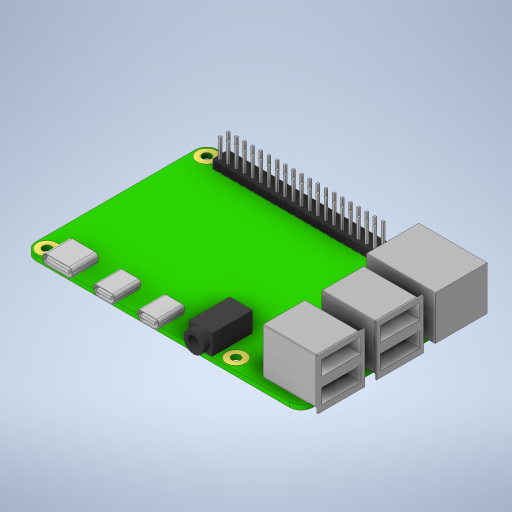
# Autodesk Inventor part: raspberry
Saved by Autodesk Inventor 2023.1 (Build 271208000, 208)
## iProperties
Created: 2022-05-23
Part Number: raspberry
Material: 일반
Document SubType Name: Modeling
Designer: fly01
Density: 1 g/cm^3
Appearance: 기본값
Author: fly01
Autodesk Inventor part; units mm, degrees
ref_plane "YZ Plane" through (0, 0, 0) normal (1, 0, 0) x (0, 1, 0)
ref_plane "XZ Plane" through (0, 0, 0) normal (0, 1, 0) x (-1, 0, 0)
ref_plane "XY Plane" through (0, 0, 0) normal (0, 0, 1) x (1, 0, 0)
sketch "스케치1" plane through (0, 0, 0) normal (0, 0, 1) x (1, 0, 0)
  line L0 (-39, 28) -> (39, 28)
  line L1 (42.5, 24.5) -> (42.5, -24.5)
  line L2 (39, -28) -> (-39, -28)
  line L3 (-42.5, -24.5) -> (-42.5, 24.5)
  line L4 (-42.5, 28) -> (42.5, -28) construction
  line L5 (42.5, 28) -> (-42.5, -28) construction
  circle A0 centre (-39, 24.5) radius 1.35
  circle A1 centre (-39, 24.5) radius 3
  line L6 (0, 0) -> (24.8557, 0)
  arc A2 (-39, 28) -> (-42.5, 24.5) centre (-39, 24.5) ccw
  circle A3 centre (19, 24.5) radius 3
  circle A4 centre (19, 24.5) radius 1.35
  circle A5 centre (-39, -24.5) radius 1.35
  circle A6 centre (-39, -24.5) radius 3
  circle A7 centre (19, -24.5) radius 3
  circle A8 centre (19, -24.5) radius 1.35
  arc A9 (-42.5, -24.5) -> (-39, -28) centre (-39, -24.5) ccw
  arc A10 (39, -28) -> (42.5, -24.5) centre (39, -24.5) ccw
  arc A11 (42.5, 24.5) -> (39, 28) centre (39, 24.5) ccw
  dimension "d0" = 85
  dimension "d1" = 56
  dimension "d2" = 2.7
  dimension "d3" = 6
  dimension "d5" = 3.5
  dimension "d6" = 3.5
  dimension "d7" = 3.5
  dimension "d10" = 58
  dimension "d15" = 3.5
  constraints: 14 end point, 12 centre point, 8 point on circle, 8 point on line, 8 tangent, 4 coincident, 4 symmetric about line, 3 horizontal, 2 equal radius, 2 midpoint, 2 parallel, 1 perpendicular, 8 other
  measures "d0" distance of L4.start L5.start
  measures "d1" distance of L5.start L4.end
  measures "d2" diameter of A0
  measures "d3" diameter of A1
  measures "d5" distance from line of L0 A0.centre
  measures "d6" distance from line of L3 A0.centre
  measures "d7" radius of A2
  measures "d10" distance of A1.centre A3.centre
  measures "d15" radius of A9
extrude "돌출1" add sketch "스케치1" against normal blind 1.5 contours L0 A11 L1 A10 L2 A9 L3 A2
extrude "돌출2" add sketch "스케치1" against normal blind 1.51 contours A1 | A3 | A6 | A7
sketch "스케치2" plane through (0, 0, -1.5) normal (0, 0, -1) x (-1, 0, 0)
  line L0 (-24.8, -25.75) -> (-45.8, -25.75)
  line L1 (-45.8, -25.75) -> (-45.8, -9.75)
  line L2 (-45.8, -9.75) -> (-24.8, -9.75)
  line L3 (-24.8, -9.75) -> (-24.8, -25.75)
  line L4 (-24.8, -25.75) -> (-45.8, -9.75) construction
  line L5 (-45.8, -25.75) -> (-24.8, -9.75) construction
  line L6 (-28.3, -5.5) -> (-45.8, -5.5)
  line L7 (-45.8, -5.5) -> (-45.8, 7.5)
  line L8 (-45.8, 7.5) -> (-28.3, 7.5)
  line L9 (-28.3, 7.5) -> (-28.3, -5.5)
  line L10 (-28.3, -5.5) -> (-45.8, 7.5) construction
  line L11 (-45.8, -5.5) -> (-28.3, 7.5) construction
  line L12 (-28.3, 12.5) -> (-45.8, 12.5)
  line L13 (-45.8, 12.5) -> (-45.8, 25.5)
  line L14 (-45.8, 25.5) -> (-28.3, 25.5)
  line L15 (-28.3, 25.5) -> (-28.3, 12.5)
  line L16 (-28.3, 12.5) -> (-45.8, 25.5) construction
  line L17 (-45.8, 12.5) -> (-28.3, 25.5) construction
  line L18 (39, 28) -> (-39, 28) projected
  line L19 (-42.5, 24.5) -> (-42.5, -24.5) projected
  point P0 (0, 0)
  point P1 (-35.3, -17.75)
  point P2 (-37.05, 1)
  point P3 (-37.05, 19)
  dimension "d20" = 45.75
  dimension "d21" = 27
  dimension "d22" = 9
  dimension "d23" = 16
  dimension "d24" = 21
  dimension "d25" = 13
  dimension "d26" = 17.5
  dimension "d27" = 13
  dimension "d28" = 17.5
  dimension "d29" = 3.3
  constraints: 36 end point, 6 midpoint, 6 parallel, 3 horizontal, 3 perpendicular, 2 point on line
  measures "d20" distance from line of L18 point (-35.3, -17.75)
  measures "d21" distance from line of L18 point (-37.05, 1)
  measures "d22" distance from line of L18 point (-37.05, 19)
  measures "d23" distance between parallel lines of L2 L0
  measures "d24" distance of L0.start L0.end
  measures "d25" distance of L6.end L7.end
  measures "d26" distance of L6.start L6.end
  measures "d27" distance of L12.end L13.end
  measures "d28" distance of L12.start L12.end
  measures "d29" distance between parallel lines of L19 L13
extrude "돌출3" add sketch "스케치2" along normal blind 13.5 contours L0 L1 L2 L3
extrude "돌출4" add sketch "스케치2" along normal blind 14 contours L6 L19 L8 L9 | L6 L7 L8 L19 | L12 L13 L14 L15
sketch "스케치3" plane through (45.8, 12.5, -1.5) normal (1, 0, 0) x (0, 0, -1)
  line L0 (0, 13) -> (0, 0) projected
  line L1 (0, 0) -> (14, 0) projected
  line L2 (14, 13) -> (14, 0) projected
  line L3 (0, 13) -> (14, 13) projected
  line L4 (0, -5) -> (0, -18) projected
  line L5 (0, -18) -> (14, -18) projected
  line L6 (14, -5) -> (14, -18) projected
  line L7 (0, -5) -> (14, -5) projected
  line L8 (14.7, -0.7) -> (-0.7, -0.7)
  line L9 (-0.7, -0.7) -> (-0.7, 13.7)
  line L10 (-0.7, 13.7) -> (14.7, 13.7)
  line L11 (14.7, 13.7) -> (14.7, -0.7)
  line L12 (14.7, -18.7) -> (-0.7, -18.7)
  line L13 (-0.7, -18.7) -> (-0.7, -4.3)
  line L14 (-0.7, -4.3) -> (14.7, -4.3)
  line L15 (14.7, -4.3) -> (14.7, -18.7)
  point P0 (-1.5, -12.5)
  dimension "d34" = 0.7
  dimension "d35" = 0.7
  constraints: 16 end point, 6 other
  measures "d34" distance between parallel lines of L2 L11
  measures "d35" distance between parallel lines of L6 L15
extrude "돌출5" add sketch "스케치3" against normal blind 0.3 contours L3 L2 L1 L0 | L7 L6 L5 L4 | L8 L9 L10 L11 | L12 L13 L14 L15
fillet "모깎기1" radius 0.2 8 edges at (36.9, 25.5, -15.5) (36.9, 12.5, -15.5) (36.9, 7.5, -15.5) (36.9, -5.5, -15.5) (44, -5.5, -1.5) (44, 7.5, -1.5) (44, 12.5, -1.5) (43.9271, 25.5, -1.5)
fillet "모깎기2" radius 1 16 edges at (45.5, -5.4414, -15.4414) (45.5, -5.5, -8.5) (45.5, -5.4414, -1.5586) (45.5, 1, -1.5) (45.5, 7.4414, -1.5586) (45.5, 7.5, -8.5) (45.5, 7.4414, -15.4414) (45.5, 1, -15.5) (45.5, 12.5586, -15.4414) (45.5, 12.5, -8.5) (45.5, 12.5586, -1.5586) (45.5, 19, -1.5) (45.5, 25.4414, -1.5586) (45.5, 25.5, -8.5) (45.5, 25.4414, -15.4414) (45.5, 19, -15.5)
sketch "스케치4" plane through (0, 0, -1.5) normal (0, 0, -1) x (-1, 0, 0)
  line L0 (35.8, 21) -> (26.8, 21)
  line L1 (26.8, 21) -> (26.8, 29)
  line L2 (26.8, 29) -> (35.8, 29)
  line L3 (35.8, 29) -> (35.8, 21)
  line L4 (35.8, 21) -> (26.8, 29) construction
  line L5 (26.8, 21) -> (35.8, 29) construction
  circle A0 centre (39, 24.5) radius 1.35 projected
  line L6 (39, 28) -> (-39, 28) projected
  point P0 (0, 0)
  point P1 (31.3, 25)
  dimension "d40" = 9
  dimension "d41" = 8
  dimension "d42" = 7.7
  dimension "d43" = 1
  constraints: 12 end point, 2 midpoint, 2 parallel, 1 horizontal, 1 perpendicular
  measures "d40" distance of L1.end L2.end
  measures "d41" distance of L0.end L1.end
  measures "d42" horizontal distance of point (31.3, 25) A0.centre
  measures "d43" distance between parallel lines of L6 L2
extrude "돌출6" add sketch "스케치4" along normal blind 3 contours L0 L1 L6 L3 | L6 L1 L2 L3
sketch "스케치5" plane through (-35.8, 29, -1.5) normal (0, 1, 0) x (1, 0, 0)
  line L0 (0, 0) -> (0, 3) projected
  line L1 (1, 3) -> (8, 3)
  line L2 (9, 2) -> (9, 1)
  line L3 (8, 0) -> (1, 0)
  line L4 (0, 1) -> (0, 2)
  arc A0 (1, 3) -> (0, 2) centre (1, 2) ccw
  arc A1 (0, 1) -> (1, 0) centre (1, 1) ccw
  arc A2 (8, 0) -> (9, 1) centre (8, 1) ccw
  arc A3 (9, 2) -> (8, 3) centre (8, 2) ccw
  line L5 (0, 3) -> (9, 3)
  line L6 (9, 3) -> (9, 0)
  line L7 (9, 0) -> (0, 0)
  line L8 (0, 0) -> (0, 3)
  line L9 (1, 2) -> (8, 2)
  line L10 (8, 2) -> (8, 1)
  line L11 (8, 1) -> (1, 1)
  line L12 (1, 1) -> (1, 2)
  line L13 (8, 2.8) -> (1, 2.8)
  arc A4 (1, 2.8) -> (0.2, 2) centre (1, 2) ccw
  line L14 (0.2, 2) -> (0.2, 1)
  arc A5 (0.2, 1) -> (1, 0.2) centre (1, 1) ccw
  line L15 (1, 0.2) -> (8, 0.2)
  arc A6 (8, 0.2) -> (8.8, 1) centre (8, 1) ccw
  line L16 (8.8, 1) -> (8.8, 2)
  arc A7 (8.8, 2) -> (8, 2.8) centre (8, 2) ccw
  point P0 (35.8, -1.5)
  point P1 (8, 0)
  point P2 (9, 1)
  point P3 (9, 2)
  point P4 (8, 3)
  point P5 (1, 3)
  point P6 (0, 2)
  point P7 (1, 0)
  point P8 (0, 1)
  dimension "d46" = 1
  dimension "d49" = 0.2
  constraints: 32 end point, 16 point on circle, 8 centre point, 8 parallel, 8 tangent, 4 perpendicular, 4 point on line, 3 equal radius, 3 horizontal, 7 other
  measures "d46" radius of A0
  measures "d49" distance between parallel lines of L1 L13
extrude "돌출7" cut sketch "스케치5" against normal blind 8 contours L0 A1 L7 | L0 L5 A0 | A2 L6 L7 | L5 L6 A3
extrude "돌출8" cut sketch "스케치5" against normal blind 7 contours A7 L16 A6 L15 A5 L14 A4 L13
sketch "스케치6" plane through (0, 0, -1.5) normal (0, 0, -1) x (-1, 0, 0)
  line L0 (19.75, 21.5) -> (13.25, 21.5)
  line L1 (13.25, 21.5) -> (13.25, 29.5)
  line L2 (13.25, 29.5) -> (19.75, 29.5)
  line L3 (19.75, 29.5) -> (19.75, 21.5)
  line L4 (19.75, 21.5) -> (13.25, 29.5) construction
  line L5 (13.25, 21.5) -> (19.75, 29.5) construction
  line L6 (34.8, 21) -> (27.8, 21) projected
  line L7 (31.3, 21) -> (31.3, 13.0642)
  line L8 (27.8, 28) -> (-39, 28) projected
  point P0 (0, 0)
  point P1 (16.5, 25.5)
  dimension "d52" = 14.8
  dimension "d53" = 1.5
  dimension "d54" = 8
  dimension "d55" = 6.5
  constraints: 14 end point, 3 midpoint, 2 parallel, 1 horizontal, 1 perpendicular, 1 vertical
  measures "d52" distance from line of L7 point (16.5, 25.5)
  measures "d53" distance between parallel lines of L8 L2
  measures "d54" distance of L0.end L1.end
  measures "d55" distance of L0.start L0.end
extrude "돌출9" add sketch "스케치6" along normal blind 3
sketch "스케치7" plane through (-19.75, 29.5, -1.5) normal (0, 1, 0) x (1, 0, 0)
  line L0 (0, 0) -> (6.5, 0) projected
  line L1 (6.5, 0) -> (6.5, 3) projected
  line L2 (0, 3) -> (6.5, 3) projected
  line L3 (0, 0) -> (0, 3) projected
  line L4 (0, 0) -> (0, 3) projected
  line L5 (0.7, 3) -> (5.8, 3)
  line L6 (6.5, 2.3) -> (6.5, 1.6348)
  line L7 (5.4261, 0) -> (1.0739, 0)
  line L8 (0, 1.6348) -> (0, 2.3)
  line L9 (0.0501, 1.3748) -> (0.424, 0.44)
  line L10 (6.4499, 1.3748) -> (6.076, 0.44)
  arc A0 (0.424, 0.44) -> (1.0739, 0) centre (1.0739, 0.7) ccw
  arc A1 (0, 1.6348) -> (0.0501, 1.3748) centre (0.7, 1.6348) ccw
  arc A2 (5.4261, 0) -> (6.076, 0.44) centre (5.4261, 0.7) ccw
  arc A3 (6.4499, 1.3748) -> (6.5, 1.6348) centre (5.8, 1.6348) ccw
  arc A4 (6.5, 2.3) -> (5.8, 3) centre (5.8, 2.3) ccw
  arc A5 (0.7, 3) -> (0, 2.3) centre (0.7, 2.3) ccw
  line L11 (0.2, 2.3) -> (0.2, 1.6348)
  arc A6 (0.2, 1.6348) -> (0.2358, 1.4491) centre (0.7, 1.6348) ccw
  line L12 (0.2358, 1.4491) -> (0.6097, 0.5143)
  arc A7 (0.6097, 0.5143) -> (1.0739, 0.2) centre (1.0739, 0.7) ccw
  line L13 (1.0739, 0.2) -> (5.4261, 0.2)
  arc A8 (5.4261, 0.2) -> (5.8903, 0.5143) centre (5.4261, 0.7) ccw
  line L14 (5.8903, 0.5143) -> (6.2642, 1.4491)
  arc A9 (6.2642, 1.4491) -> (6.3, 1.6348) centre (5.8, 1.6348) ccw
  line L15 (6.3, 1.6348) -> (6.3, 2.3)
  arc A10 (6.3, 2.3) -> (5.8, 2.8) centre (5.8, 2.3) ccw
  line L16 (5.8, 2.8) -> (0.7, 2.8)
  arc A11 (0.7, 2.8) -> (0.2, 2.3) centre (0.7, 2.3) ccw
  line L17 (1.0733, 1.9674) -> (5.3358, 1.9674)
  line L18 (5.3358, 1.9674) -> (5.3358, 1.2025)
  line L19 (5.3358, 1.2025) -> (1.0733, 1.2025)
  line L20 (1.0733, 1.2025) -> (1.0733, 1.9674)
  point P0 (19.75, -1.5)
  point P1 (0, 1.5)
  point P2 (0.6, 0)
  point P3 (6.5, 1.5)
  point P4 (5.9, 0)
  point P5 (0, 2.3)
  point P6 (0.7, 3)
  point P7 (0, 1.6348)
  point P8 (6.5, 1.6348)
  point P9 (5.8, 3)
  dimension "d58" = 1.5
  dimension "d59" = 0.6
  dimension "d60" = 1.5
  dimension "d61" = 0.6
  dimension "d62" = 0.7
  dimension "d63" = 0.2
  constraints: 32 end point, 24 point on circle, 14 point on line, 12 centre point, 12 tangent, 6 parallel, 5 equal radius, 3 perpendicular, 2 horizontal, 11 other
  measures "d58" distance of point (0, 1.5) point (0, 0)
  measures "d59" distance of point (0.6, 0) point (0, 0)
  measures "d60" distance of point (6.5, 1.5) L0.end
  measures "d61" distance of point (5.9, 0) L0.end
  measures "d62" radius of A0
  measures "d63" radial gap between concentric circles of A5 A11
extrude "돌출10" cut sketch "스케치7" against normal blind 8 contours L3 A1 L9 A0 L0 | A2 L10 A3 L1 L0 | L3 L2 A5 | L2 L1 A4
extrude "돌출11" cut sketch "스케치7" against normal blind 7 contours A11 L16 A10 L15 A9 L14 A8 L13 A7 L12 A6 L11
pattern_linear "직사각형 패턴1" count 2 spacing 13.5 along (1, 0, 0) of "돌출10", "돌출11", "돌출9"
sketch "스케치8" plane through (0, 0, -1.5) normal (0, 0, -1) x (-1, 0, 0)
  line L0 (-15, -27.0906) -> (-15, -22.0906)
  line L1 (35, -22.0906) -> (35, -26.7906)
  line L2 (10, -27.0906) -> (10, -24.2193)
  circle A0 centre (-19, -24.5) radius 1.35 projected
  line L3 (34.7, -27.0906) -> (32.8, -27.0906)
  line L4 (32.5, -26.7906) -> (32.5, -22.3906)
  line L5 (32.8, -22.0906) -> (34.7, -22.0906)
  line L6 (35, -22.3906) -> (35, -27.0906)
  line L7 (32.8, -22.0906) -> (32.5, -22.3906)
  line L8 (32.5, -26.7906) -> (32.8, -27.0906)
  line L9 (34.7, -27.0906) -> (35, -26.7906)
  line L10 (34.7, -22.0906) -> (35, -22.3906)
  point P0 (0, 0)
  point P1 (32.5, -22.0906)
  point P2 (32.5, -27.0906)
  point P3 (35, -24.5906)
  dimension "d71" = 29
  dimension "d72" = 50
  dimension "d73" = 5
  dimension "d74" = 2.5
  dimension "d75" = 5
  dimension "d78" = 0.3
  dimension "d79" = 0.3
  dimension "d80" = 0.3
  dimension "d81" = 0.3
  dimension "d82" = 0.3
  dimension "d83" = 0.3
  dimension "d84" = 0.3
  dimension "d85" = 0.3
  constraints: 22 end point, 8 point on line, 3 parallel, 1 horizontal, 1 perpendicular, 1 vertical
  measures "d71" distance from line of L2 A0.centre
  measures "d72" distance of L0.end L1.start
  measures "d73" distance of L0.start L0.end
  measures "d74" distance of point (32.5, -22.091) point (35, -22.091)
  measures "d75" distance of point (32.5, -27.091) point (32.5, -22.091)
  measures "d78" distance of L5.start point (32.5, -22.091)
  measures "d79" distance of L4.end point (32.5, -22.091)
  measures "d80" distance of L4.start point (32.5, -27.091)
  measures "d81" distance of L3.end point (32.5, -27.091)
  measures "d82" distance of L3.start L6.end
  measures "d83" distance of L1.end L6.end
  measures "d84" distance of L5.end point (35, -22.091)
  measures "d85" distance of L6.start point (35, -22.091)
extrude "돌출12" add sketch "스케치8" along normal blind 2.5 contours L1 L9 L3 L8 L4 L7 L5 L10
sketch "스케치9" plane through (0, 0, -4) normal (0, 0, -1) x (-1, 0, 0)
  line L0 (32.8, -22.0906) -> (32.5, -22.3906) projected
  line L1 (32.5, -22.3906) -> (32.5, -26.7906) projected
  line L2 (32.5, -26.7906) -> (32.8, -27.0906) projected
  line L3 (32.8, -27.0906) -> (34.7, -27.0906) projected
  line L4 (34.7, -27.0906) -> (35, -26.7906) projected
  line L5 (35, -26.7906) -> (35, -22.3906) projected
  line L6 (35, -22.3906) -> (34.7, -22.0906) projected
  line L7 (34.7, -22.0906) -> (32.8, -22.0906) projected
  line L8 (34.7, -27.0906) -> (32.8, -27.0906) projected
  line L9 (32.8, -22.0906) -> (34.7, -22.0906) projected
  line L10 (34.05, -26.1406) -> (33.45, -26.1406)
  line L11 (33.45, -26.1406) -> (33.45, -25.5406)
  line L12 (33.45, -25.5406) -> (34.05, -25.5406)
  line L13 (34.05, -25.5406) -> (34.05, -26.1406)
  line L14 (34.05, -26.1406) -> (33.45, -25.5406) construction
  line L15 (33.45, -26.1406) -> (34.05, -25.5406) construction
  line L16 (35, -22.3906) -> (35, -26.7906) projected
  line L17 (35, -24.5906) -> (32.5, -24.5906) construction
  line L18 (33.75, -27.0906) -> (33.75, -24.5906) construction
  line L19 (34.05, -23.0406) -> (33.45, -23.0406)
  line L20 (33.45, -23.6406) -> (34.05, -23.6406)
  line L21 (34.05, -23.6406) -> (34.05, -23.0406)
  line L22 (33.45, -23.6406) -> (33.45, -23.0406)
  point P0 (0, 0)
  point P1 (33.75, -25.8406)
  point P2 (33.75, -25.8406)
  dimension "d86" = 0.6
  dimension "d87" = 0.6
  constraints: 24 end point, 8 midpoint, 4 symmetric about line, 2 parallel, 1 horizontal, 1 perpendicular, 1 vertical
  measures "d86" distance of L11.end L12.end
  measures "d87" distance of L10.end L11.end
extrude "돌출13" add sketch "스케치9" along normal blind 6 contours L10 L11 L12 L13 | L21 L20 L22 L19
chamfer "모따기1" distance 0.1 angle 45 8 edges at (-32.65, -22.2406, -4) (-32.5, -24.5906, -4) (-33.75, -22.0906, -4) (-34.85, -22.2406, -4) (-35, -24.5906, -4) (-34.85, -26.9406, -4) (-33.75, -27.0906, -4) (-32.65, -26.9406, -4)
pattern_linear "직사각형 패턴2" count 20 spacing 2.5 along (1, 0, 0) of "돌출13", "돌출12", "모따기1"
sketch "스케치11" plane through (-39, 28, 0) normal (0, 1, 0) x (1, 0, 0)
  line L0 (78, 1.5) -> (0, 1.5) projected
  line L1 (47.05, 1.5) -> (54.05, 1.5)
  line L2 (54.05, 1.5) -> (54.05, 7.7)
  line L3 (54.05, 7.7) -> (47.05, 7.7)
  line L4 (47.05, 7.7) -> (47.05, 1.5)
  line L5 (39.25, 3.1348) -> (39.25, 3.8) projected
  line L6 (47.05, 4.6) -> (54.05, 4.6)
  line L7 (50.55, 4) -> (50.55, 10) projected
  circle A0 centre (50.55, 4.6) radius 3.1
  point P0 (39, 0)
  point P1 (50.55, 7.7)
  point P2 (50.55, 1.5)
  dimension "d96" = 7.8
  dimension "d97" = 6.2
  dimension "d98" = 7
  constraints: 10 end point, 3 midpoint, 2 parallel, 2 point on line, 1 centre point, 1 horizontal, 1 perpendicular
  measures "d96" distance between parallel lines of L4 L5
  measures "d97" distance of L1.end L2.end
  measures "d98" distance of L2.end L3.end
extrude "돌출14" add sketch "스케치11" against normal blind 12.5
extrude "돌출15" add sketch "스케치11" along normal blind 2.08 contours A0 L6 | A0 L7 L6 | L6 L7 A0
sketch "스케치12" plane through (11.55, 30.08, -4.6) normal (0, 1, 0) x (1, 0, 0)
  line L0 (0, -0.6) -> (0, 5.4) projected
  circle A0 centre (0, 0.0034) radius 1.835
  point P0 (-11.55, -4.6)
  dimension "d104" = 3.67
  constraints: 1 centre point, 1 point on line
  measures "d104" diameter of A0
extrude "돌출16" cut sketch "스케치12" against normal blind 17.17
extrude "돌출17" cut sketch "스케치11" against normal blind 0.1 contours L0 A0 L6 L2 | L0 L4 L6 A0 | L6 A0 L3 L2 | L6 L4 L3 A0
sketch "스케치14" plane through (45.8, -6.2, -0.8) normal (1, 0, 0) x (0, 0, -1)
  line L0 (13.9, 13.2) -> (9.4, 13.2)
  line L1 (9.4, 13.2) -> (9.4, 1.2)
  line L2 (9.4, 1.2) -> (13.9, 1.2)
  line L3 (13.9, 1.2) -> (13.9, 13.2)
  line L4 (15.4, 0) -> (15.4, 14.4) projected
  point P0 (-0.8, 6.2)
  point P1 (13.9, 7.2)
  point P2 (15.4, 7.2)
  dimension "d109" = 12
  dimension "d110" = 4.5
  dimension "d111" = 1.5
  constraints: 8 end point, 2 midpoint, 2 parallel, 1 horizontal, 1 horizontal alignment, 1 perpendicular
  measures "d109" distance of L2.end L0.start
  measures "d110" distance of L1.end L2.end
  measures "d111" distance between parallel lines of L4 L3
extrude "돌출18" cut sketch "스케치14" against normal blind 15
pattern_linear "직사각형 패턴3" count 2 spacing 7.5 along (0, 0, 1) count 2 spacing 18 along (0, 1, 0) of "돌출18"
equation "\"d60\" = d58"
equation "\"d61\" = d59"
equation "\"d79\" = d78"
equation "\"d80\" = d78"
equation "\"d81\" = d80"
equation "\"d82\" = d78"
equation "\"d83\" = d82"
equation "\"d84\" = d78"
equation "\"d85\" = d84"
